Autodesk Fusion 360 part; units mm, degrees
(part 6 of 6)
  spline S1882 degree 3 poles (-65.5883, -15.6255) (-65.5532, -15.6205) (-65.5182, -15.6155) (-65.4821, -15.6104) knots 0 0 0 0 1 1 1 1
  spline S1883 degree 3 poles (-65.4821, -15.6104) (-65.2398, -15.5688) (-65.2398, -15.5688) (-65.135, -15.4302) knots 0 0 0 0 1 1 1 1
  spline S1884 degree 3 poles (-65.135, -15.4302) (-65.0343, -15.1397) (-65.091, -14.7914) (-65.1957, -14.5049) knots 0 0 0 0 1 1 1 1
  spline S1885 degree 3 poles (-65.1957, -14.5049) (-65.2987, -14.382) (-65.405, -14.3558) (-65.5585, -14.321) knots 0 0 0 0 1 1 1 1
  spline S1886 degree 3 poles (-65.5585, -14.321) (-65.627, -14.3026) (-65.627, -14.3026) (-65.6969, -14.2838) knots 0 0 0 0 1 1 1 1
  spline S1887 degree 3 poles (-65.6969, -14.2838) (-65.9478, -14.2203) (-66.2008, -14.1721) (-66.4553, -14.1254) knots 0 0 0 0 1 1 1 1
  spline S1888 degree 3 poles (-66.4553, -14.1254) (-66.8857, -14.0468) (-66.8857, -14.0468) (-67.2221, -13.7882) knots 0 0 0 0 1 1 1 1
  spline S1889 degree 3 poles (-67.2221, -13.7882) (-67.2338, -13.7221) (-67.2455, -13.656) (-67.2575, -13.5879) knots 0 0 0 0 1 1 1 1
  spline S1890 degree 3 poles (-67.2575, -13.5879) (-67.0063, -13.5436) (-66.7551, -13.4993) (-66.4963, -13.4537) knots 0 0 0 0 1 1 1 1
  spline S1891 degree 3 poles (-66.4963, -13.4537) (-66.4997, -13.3198) (-66.5032, -13.186) (-66.5066, -13.0521) knots 0 0 0 0 1 1 1 1
  spline S1892 degree 3 poles (-66.5066, -13.0521) (-66.5107, -12.9269) (-66.5107, -12.9269) (-66.4985, -12.8356) knots 0 0 0 0 1 1 1 1
  spline S1893 degree 3 poles (-66.4985, -12.8356) (-66.495, -12.7075) (-66.5308, -12.5902) (-66.5595, -12.4657) knots 0 0 0 0 1 1 1 1
  spline S1894 degree 3 poles (-66.5595, -12.4657) (-66.6167, -12.177) (-66.5859, -11.9942) (-66.4254, -11.7476) knots 0 0 0 0 1 1 1 1
  spline S1895 degree 3 poles (-66.4254, -11.7476) (-66.3616, -11.6547) (-66.2962, -11.5632) (-66.2298, -11.472) knots 0 0 0 0 1 1 1 1
  spline S1896 degree 3 poles (-66.2298, -11.472) (-66.0403, -11.1911) (-65.8738, -10.8747) (-65.8549, -10.5317) knots 0 0 0 0 1 1 1 1
  spline S1897 degree 3 poles (-65.8549, -10.5317) (-65.8517, -10.4954) (-65.8484, -10.4591) (-65.8451, -10.4217) knots 0 0 0 0 1 1 1 1
  spline S1898 degree 3 poles (-65.8451, -10.4217) (-65.8423, -10.2464) (-65.8489, -10.1305) (-65.972, -9.9994) knots 0 0 0 0 1 1 1 1
  spline S1899 degree 3 poles (-65.972, -9.9994) (-66.0832, -9.9196) (-66.1966, -9.8527) (-66.3167, -9.787) knots 0 0 0 0 1 1 1 1
  spline S1900 degree 3 poles (-66.3167, -9.787) (-66.3519, -9.766) (-66.3871, -9.745) (-66.4234, -9.7234) knots 0 0 0 0 1 1 1 1
  spline S1901 degree 3 poles (-66.4234, -9.7234) (-67.0299, -9.3691) (-67.6639, -9.045) (-68.3125, -8.7758) knots 0 0 0 0 1 1 1 1
  spline S1902 degree 3 poles (-68.3125, -8.7758) (-68.3713, -8.7504) (-68.43, -8.7249) (-68.4886, -8.6994) knots 0 0 0 0 1 1 1 1
  spline S1903 degree 3 poles (-68.4886, -8.6994) (-68.8092, -8.5606) (-69.1312, -8.4289) (-69.4605, -8.3121) knots 0 0 0 0 1 1 1 1
  spline S1904 degree 3 poles (-69.4605, -8.3121) (-69.4898, -8.3016) (-69.519, -8.2912) (-69.5492, -8.2804) knots 0 0 0 0 1 1 1 1
  spline S1905 degree 3 poles (-69.5492, -8.2804) (-69.8961, -8.1602) (-70.2263, -8.1917) (-70.5689, -8.3301) knots 0 0 0 0 1 1 1 1
  spline S1906 degree 3 poles (-70.5689, -8.3301) (-71.0757, -8.6136) (-71.3065, -9.1813) (-71.5588, -9.6756) knots 0 0 0 0 1 1 1 1
  spline S1907 degree 3 poles (-71.5588, -9.6756) (-71.6206, -9.7962) (-71.6842, -9.9157) (-71.7488, -10.0348) knots 0 0 0 0 1 1 1 1
  spline S1908 degree 3 poles (-71.7488, -10.0348) (-71.7661, -10.0671) (-71.7835, -10.0994) (-71.8014, -10.1327) knots 0 0 0 0 1 1 1 1
  spline S1909 degree 3 poles (-71.8014, -10.1327) (-71.857, -10.2311) (-71.857, -10.2311) (-71.9354, -10.3313) knots 0 0 0 0 1 1 1 1
  spline S1910 degree 3 poles (-71.9354, -10.3313) (-72.0284, -10.4725) (-72.0876, -10.6124) (-72.1415, -10.7713) knots 0 0 0 0 1 1 1 1
  spline S1911 degree 3 poles (-72.1415, -10.7713) (-72.152, -10.8016) (-72.1624, -10.8319) (-72.1732, -10.8631) knots 0 0 0 0 1 1 1 1
  spline S1912 degree 3 poles (-72.1732, -10.8631) (-72.3084, -11.2678) (-72.4026, -11.6835) (-72.5002, -12.0984) knots 0 0 0 0 1 1 1 1
  spline S1913 degree 3 poles (-72.5002, -12.0984) (-72.6463, -13.0231) (-72.6463, -13.0231) (-73.0404, -13.8227) knots 0 0 0 0 1 1 1 1
  spline S1914 degree 3 poles (-73.0404, -13.8227) (-73.1439, -13.8634) (-73.2458, -13.891) (-73.3538, -13.9193) knots 0 0 0 0 1 1 1 1
  spline S1915 degree 3 poles (-73.3538, -13.9193) (-73.3286, -13.9617) (-73.3035, -14.0041) (-73.2775, -14.0477) knots 0 0 0 0 1 1 1 1
  spline S1916 degree 3 poles (-73.2775, -14.0477) (-73.1826, -14.2076) (-73.0879, -14.3676) (-72.9931, -14.5276) knots 0 0 0 0 1 1 1 1
  spline S1917 degree 3 poles (-72.9931, -14.5276) (-72.9524, -14.5964) (-72.9117, -14.6651) (-72.8709, -14.7338) knots 0 0 0 0 1 1 1 1
  spline S1918 degree 3 poles (-72.8709, -14.7338) (-72.4098, -15.5103) (-71.9883, -16.2311) (-71.8222, -17.1294) knots 0 0 0 0 1 1 1 1
  spline S1919 degree 3 poles (-71.8222, -17.1294) (-71.814, -17.1724) (-71.8059, -17.2155) (-71.7975, -17.2598) knots 0 0 0 0 1 1 1 1
  spline S1920 degree 3 poles (-71.7975, -17.2598) (-71.7166, -17.7347) (-71.7778, -18.178) (-71.8669, -18.6475) knots 0 0 0 0 1 1 1 1
  spline S1921 degree 3 poles (-71.8669, -18.6475) (-71.8753, -18.6921) (-71.8838, -18.7366) (-71.8925, -18.7825) knots 0 0 0 0 1 1 1 1
  spline S1922 degree 3 poles (-71.8925, -18.7825) (-71.9993, -19.3246) (-72.1479, -19.8096) (-72.438, -20.2844) knots 0 0 0 0 1 1 1 1
  spline S1923 degree 3 poles (-72.438, -20.2844) (-72.4548, -20.3194) (-72.4715, -20.3544) (-72.4888, -20.3905) knots 0 0 0 0 1 1 1 1
  spline S1924 degree 3 poles (-72.4888, -20.3905) (-72.5833, -20.565) (-72.6683, -20.6588) (-72.859, -20.7171) knots 0 0 0 0 1 1 1 1
  spline S1925 degree 3 poles (-72.859, -20.7171) (-73.0033, -20.754) (-73.1488, -20.7807) (-73.2957, -20.8049) knots 0 0 0 0 1 1 1 1
  spline S1926 degree 3 poles (-73.2957, -20.8049) (-73.376, -20.8215) (-73.376, -20.8215) (-73.5135, -20.874) knots 0 0 0 0 1 1 1 1
  spline S1927 degree 3 poles (-73.5135, -20.874) (-73.6824, -20.92) (-73.8082, -20.8944) (-73.9726, -20.8493) knots 0 0 0 0 1 1 1 1
  spline S1928 degree 3 poles (-73.9726, -20.8493) (-74.0026, -20.8414) (-74.0327, -20.8335) (-74.0636, -20.8253) knots 0 0 0 0 1 1 1 1
  spline S1929 degree 3 poles (-74.0636, -20.8253) (-75.2169, -20.508) (-75.8729, -19.7935) (-76.5711, -18.8652) knots 0 0 0 0 1 1 1 1
  spline S1930 degree 3 poles (-76.5711, -18.8652) (-76.6006, -18.8261) (-76.6006, -18.8261) (-76.6307, -18.7863) knots 0 0 0 0 1 1 1 1
  spline S1931 degree 3 poles (-76.6307, -18.7863) (-76.8351, -18.5226) (-76.8351, -18.5226) (-77.0117, -18.2406) knots 0 0 0 0 1 1 1 1
  spline S1932 degree 3 poles (-77.0117, -18.2406) (-77.1093, -18.214) (-77.1093, -18.214) (-77.2261, -18.1958) knots 0 0 0 0 1 1 1 1
  spline S1933 degree 3 poles (-77.2261, -18.1958) (-77.26, -18.1873) (-77.2939, -18.1788) (-77.3288, -18.17) knots 0 0 0 0 1 1 1 1
  spline S1934 degree 3 poles (-77.3288, -18.17) (-77.6049, -18.1231) (-77.8749, -18.1799) (-78.1471, -18.2291) knots 0 0 0 0 1 1 1 1
  spline S1935 degree 3 poles (-78.1471, -18.2291) (-78.1833, -18.2354) (-78.2195, -18.2416) (-78.2568, -18.248) knots 0 0 0 0 1 1 1 1
  spline S1936 degree 3 poles (-78.2568, -18.248) (-78.4722, -18.2863) (-78.6745, -18.3386) (-78.8828, -18.4053) knots 0 0 0 0 1 1 1 1
  spline S1937 degree 3 poles (-78.8828, -18.4053) (-79.2946, -18.5224) (-79.2946, -18.5224) (-79.6968, -18.4301) knots 0 0 0 0 1 1 1 1
  spline S1938 degree 3 poles (-79.6968, -18.4301) (-79.7779, -18.38) (-79.7779, -18.38) (-79.8466, -18.3274) knots 0 0 0 0 1 1 1 1
  spline S1939 degree 3 poles (-79.8466, -18.3274) (-79.8777, -18.3056) (-79.9088, -18.2839) (-79.9408, -18.2614) knots 0 0 0 0 1 1 1 1
  spline S1940 degree 3 poles (-79.9408, -18.2614) (-79.9702, -18.1606) (-79.9702, -18.1606) (-79.9867, -18.0449) knots 0 0 0 0 1 1 1 1
  spline S1941 degree 3 poles (-79.9867, -18.0449) (-79.9933, -18.0061) (-79.9999, -17.9673) (-80.0067, -17.9273) knots 0 0 0 0 1 1 1 1
  spline S1942 degree 3 poles (-80.0067, -17.9273) (-80.0235, -17.8171) (-80.0235, -17.8171) (-79.9997, -17.6935) knots 0 0 0 0 1 1 1 1
  spline S1943 degree 3 poles (-79.9997, -17.6935) (-80.0127, -17.4367) (-80.0653, -17.2516) (-80.2492, -17.0682) knots 0 0 0 0 1 1 1 1
  spline S1944 degree 3 poles (-80.2492, -17.0682) (-80.3329, -17.0032) (-80.4149, -16.9607) (-80.5111, -16.9162) knots 0 0 0 0 1 1 1 1
  spline S1945 degree 3 poles (-80.5111, -16.9162) (-80.7636, -16.7989) (-80.8627, -16.6336) (-80.9708, -16.3835) knots 0 0 0 0 1 1 1 1
  spline S1946 degree 3 poles (-80.9708, -16.3835) (-81.0257, -16.194) (-80.9508, -16.0807) (-80.843, -15.9266) knots 0 0 0 0 1 1 1 1
  spline S1947 degree 3 poles (-61.3294, -20.2671) (-61.263, -20.2962) (-61.263, -20.2962) (-61.1951, -20.326) knots 0 0 0 0 1 1 1 1
  spline S1948 degree 3 poles (-61.1951, -20.326) (-61.2348, -20.333) (-61.2744, -20.34) (-61.3153, -20.3472) knots 0 0 0 0 1 1 1 1
  spline S1949 degree 3 poles (-61.3153, -20.3472) (-61.32, -20.3207) (-61.3246, -20.2943) (-61.3294, -20.2671) knots 0 0 0 0 1 1 1 1
  spline S1950 degree 3 poles (-59.751, 10.372) (-59.6633, 10.465) (-59.5616, 10.5119) (-59.4464, 10.565) knots 0 0 0 0 1 1 1 1
  spline S1951 degree 3 poles (-59.4464, 10.565) (-59.4153, 10.5807) (-59.3843, 10.5964) (-59.3523, 10.6127) knots 0 0 0 0 1 1 1 1
  spline S1952 degree 3 poles (-59.3523, 10.6127) (-59.2858, 10.6462) (-59.219, 10.6791) (-59.152, 10.7115) knots 0 0 0 0 1 1 1 1
  spline S1953 degree 3 poles (-59.152, 10.7115) (-58.977, 10.7962) (-58.8043, 10.8855) (-58.6312, 10.9741) knots 0 0 0 0 1 1 1 1
  spline S1954 degree 3 poles (-58.6312, 10.9741) (-58.5971, 10.9914) (-58.5629, 11.0088) (-58.5277, 11.0266) knots 0 0 0 0 1 1 1 1
  spline S1955 degree 3 poles (-58.5277, 11.0266) (-57.7705, 11.4124) (-57.0352, 11.9023) (-56.4295, 12.5015) knots 0 0 0 0 1 1 1 1
  spline S1956 degree 3 poles (-56.4295, 12.5015) (-56.0056, 12.9201) (-55.4738, 13.0694) (-54.9102, 13.212) knots 0 0 0 0 1 1 1 1
  spline S1957 degree 3 poles (-54.9102, 13.212) (-54.2791, 13.3732) (-53.6906, 13.592) (-53.0958, 13.8587) knots 0 0 0 0 1 1 1 1
  spline S1958 degree 3 poles (-53.0958, 13.8587) (-52.9602, 13.9188) (-52.8245, 13.9787) (-52.6887, 14.0383) knots 0 0 0 0 1 1 1 1
  spline S1959 degree 3 poles (-52.6887, 14.0383) (-52.6043, 14.0754) (-52.52, 14.113) (-52.4359, 14.151) knots 0 0 0 0 1 1 1 1
  spline S1960 degree 3 poles (-52.4359, 14.151) (-52.3984, 14.1676) (-52.3609, 14.1843) (-52.3223, 14.2014) knots 0 0 0 0 1 1 1 1
  spline S1961 degree 3 poles (-52.3223, 14.2014) (-52.2894, 14.2163) (-52.2565, 14.2311) (-52.2226, 14.2464) knots 0 0 0 0 1 1 1 1
  spline S1962 degree 3 poles (-52.2226, 14.2464) (-52.1313, 14.2848) (-52.1313, 14.2848) (-52.0094, 14.2568) knots 0 0 0 0 1 1 1 1
  spline S1963 degree 3 poles (-52.0094, 14.2568) (-52.0534, 14.2314) (-52.0974, 14.206) (-52.1428, 14.1798) knots 0 0 0 0 1 1 1 1
  spline S1964 degree 3 poles (-52.1428, 14.1798) (-52.5791, 13.919) (-52.9072, 13.6269) (-53.2354, 13.2404) knots 0 0 0 0 1 1 1 1
  spline S1965 degree 3 poles (-53.2354, 13.2404) (-53.3211, 13.1403) (-53.4099, 13.0432) (-53.4989, 12.946) knots 0 0 0 0 1 1 1 1
  spline S1966 degree 3 poles (-53.4989, 12.946) (-53.6938, 12.7322) (-53.8771, 12.5123) (-54.0526, 12.2821) knots 0 0 0 0 1 1 1 1
  spline S1967 degree 3 poles (-54.0526, 12.2821) (-54.1106, 12.2071) (-54.1701, 12.136) (-54.233, 12.0652) knots 0 0 0 0 1 1 1 1
  spline S1968 degree 3 poles (-54.233, 12.0652) (-54.3312, 11.9443) (-54.4082, 11.8212) (-54.4872, 11.6874) knots 0 0 0 0 1 1 1 1
  spline S1969 degree 3 poles (-54.4872, 11.6874) (-54.5654, 11.5559) (-54.6458, 11.4259) (-54.7274, 11.2965) knots 0 0 0 0 1 1 1 1
  spline S1970 degree 3 poles (-54.7274, 11.2965) (-54.7428, 11.2721) (-54.7582, 11.2477) (-54.774, 11.2226) knots 0 0 0 0 1 1 1 1
  spline S1971 degree 3 poles (-54.774, 11.2226) (-54.857, 11.093) (-54.9434, 10.9736) (-55.0452, 10.8584) knots 0 0 0 0 1 1 1 1
  spline S1972 degree 3 poles (-55.0452, 10.8584) (-55.2359, 10.6313) (-55.3492, 10.3545) (-55.4744, 10.0881) knots 0 0 0 0 1 1 1 1
  spline S1973 degree 3 poles (-55.4744, 10.0881) (-55.5326, 9.9644) (-55.5924, 9.8415) (-55.6523, 9.7187) knots 0 0 0 0 1 1 1 1
  spline S1974 degree 3 poles (-55.6523, 9.7187) (-55.6804, 9.6603) (-55.6804, 9.6603) (-55.7091, 9.6007) knots 0 0 0 0 1 1 1 1
  spline S1975 degree 3 poles (-55.7091, 9.6007) (-55.7555, 9.5039) (-55.7555, 9.5039) (-55.8229, 9.4123) knots 0 0 0 0 1 1 1 1
  spline S1976 degree 3 poles (-55.8229, 9.4123) (-55.931, 9.3943) (-56.0328, 9.3834) (-56.1419, 9.3767) knots 0 0 0 0 1 1 1 1
  spline S1977 degree 3 poles (-56.1419, 9.3767) (-56.1755, 9.3747) (-56.2092, 9.3726) (-56.2439, 9.3704) knots 0 0 0 0 1 1 1 1
  spline S1978 degree 3 poles (-56.2439, 9.3704) (-56.9302, 9.336) (-57.6315, 9.3267) (-58.2906, 9.5376) knots 0 0 0 0 1 1 1 1
  spline S1979 degree 3 poles (-58.2906, 9.5376) (-58.5865, 9.6318) (-58.8906, 9.6973) (-59.1928, 9.7682) knots 0 0 0 0 1 1 1 1
  spline S1980 degree 3 poles (-59.1928, 9.7682) (-59.2522, 9.7823) (-59.3116, 9.7963) (-59.3711, 9.8104) knots 0 0 0 0 1 1 1 1
  spline S1981 degree 3 poles (-59.3711, 9.8104) (-59.5119, 9.8438) (-59.6527, 9.877) (-59.7935, 9.9101) knots 0 0 0 0 1 1 1 1
  spline S1982 degree 3 poles (-59.7935, 9.9101) (-59.8214, 10.0683) (-59.8022, 10.2204) (-59.751, 10.372) knots 0 0 0 0 1 1 1 1
  line L6 (-50.8593, 14.9966) -> (-50.9465, 15.0225)
  line L7 (-50.7862, 15.0507) -> (-50.8734, 15.0767)
  spline S1983 degree 3 poles (-29.2882, 12.6041) (-28.8697, 12.7557) (-28.5896, 12.7131) (-28.1934, 12.5283) knots 0 0 0 0 1 1 1 1
  spline S1984 degree 3 poles (-28.1934, 12.5283) (-28.0851, 12.4763) (-27.9778, 12.4225) (-27.8706, 12.3684) knots 0 0 0 0 1 1 1 1
  spline S1985 degree 3 poles (-27.8706, 12.3684) (-27.7226, 12.2949) (-27.5716, 12.228) (-27.4211, 12.1599) knots 0 0 0 0 1 1 1 1
  spline S1986 degree 3 poles (-27.4211, 12.1599) (-27.3957, 12.147) (-27.3703, 12.134) (-27.3442, 12.1207) knots 0 0 0 0 1 1 1 1
  spline S1987 degree 3 poles (-27.3442, 12.1207) (-27.3418, 12.1075) (-27.3395, 12.0943) (-27.3371, 12.0806) knots 0 0 0 0 1 1 1 1
  spline S1988 degree 3 poles (-27.3371, 12.0806) (-27.3612, 12.0758) (-27.3853, 12.071) (-27.4102, 12.0661) knots 0 0 0 0 1 1 1 1
  spline S1989 degree 3 poles (-27.4102, 12.0661) (-27.6928, 11.9997) (-27.879, 11.8794) (-28.1005, 11.6956) knots 0 0 0 0 1 1 1 1
  spline S1990 degree 3 poles (-28.1005, 11.6956) (-28.1317, 11.6706) (-28.1628, 11.6456) (-28.1949, 11.6198) knots 0 0 0 0 1 1 1 1
  spline S1991 degree 3 poles (-28.1949, 11.6198) (-28.2708, 11.5588) (-28.3462, 11.4972) (-28.4212, 11.4351) knots 0 0 0 0 1 1 1 1
  spline S1992 degree 3 poles (-28.4212, 11.4351) (-28.5203, 11.5389) (-28.5593, 11.6131) (-28.6197, 11.7409) knots 0 0 0 0 1 1 1 1
  spline S1993 degree 3 poles (-28.6197, 11.7409) (-28.7463, 11.9829) (-28.9129, 12.1609) (-29.1051, 12.3513) knots 0 0 0 0 1 1 1 1
  spline S1994 degree 3 poles (-29.1051, 12.3513) (-29.2274, 12.4594) (-29.2274, 12.4594) (-29.2882, 12.6041) knots 0 0 0 0 1 1 1 1
  spline S1995 degree 3 poles (-8.3515, -3.8776) (-8.3386, -3.8501) (-8.3257, -3.8226) (-8.3125, -3.7942) knots 0 0 0 0 1 1 1 1
  spline S1996 degree 3 poles (-8.3125, -3.7942) (-8.2806, -3.7262) (-8.2484, -3.6583) (-8.2162, -3.5904) knots 0 0 0 0 1 1 1 1
  spline S1997 degree 3 poles (-8.2162, -3.5904) (-8.1894, -3.6266) (-8.1894, -3.6266) (-8.1621, -3.6635) knots 0 0 0 0 1 1 1 1
  spline S1998 degree 3 poles (-8.1621, -3.6635) (-8.1884, -3.7667) (-8.1884, -3.7667) (-8.2348, -3.8803) knots 0 0 0 0 1 1 1 1
  spline S1999 degree 3 poles (-8.2348, -3.8803) (-8.2495, -3.919) (-8.2641, -3.9577) (-8.2792, -3.9976) knots 0 0 0 0 1 1 1 1
  spline S2000 degree 3 poles (-8.2792, -3.9976) (-8.3311, -4.105) (-8.3848, -4.1735) (-8.4708, -4.2549) knots 0 0 0 0 1 1 1 1
  spline S2001 degree 3 poles (-8.4708, -4.2549) (-8.495, -4.1179) (-8.4095, -3.9996) (-8.3515, -3.8776) knots 0 0 0 0 1 1 1 1
  spline S2002 degree 3 poles (-21.8258, -8.6338) (-21.2854, -9.6912) (-19.7141, -10.0697) (-18.6621, -10.4138) knots 0 0 0 0 1 1 1 1
  spline S2003 degree 3 poles (-18.6621, -10.4138) (-17.9941, -10.6297) (-17.3212, -10.8297) (-16.6476, -11.0274) knots 0 0 0 0 1 1 1 1
  spline S2004 degree 3 poles (-16.6476, -11.0274) (-16.588, -11.045) (-16.5284, -11.0625) (-16.4689, -11.0801) knots 0 0 0 0 1 1 1 1
  spline S2005 degree 3 poles (-16.4689, -11.0801) (-16.4402, -11.0885) (-16.4115, -11.0969) (-16.382, -11.1055) knots 0 0 0 0 1 1 1 1
  spline S2006 degree 3 poles (-16.382, -11.1055) (-16.2422, -11.1468) (-16.1039, -11.1905) (-15.9666, -11.2396) knots 0 0 0 0 1 1 1 1
  spline S2007 degree 3 poles (-15.9666, -11.2396) (-15.8908, -11.2665) (-15.8908, -11.2665) (-15.8135, -11.294) knots 0 0 0 0 1 1 1 1
  spline S2008 degree 3 poles (-15.8135, -11.294) (-15.7691, -11.3105) (-15.7248, -11.327) (-15.6791, -11.344) knots 0 0 0 0 1 1 1 1
  spline S2009 degree 3 poles (-15.6791, -11.344) (-15.5418, -11.3747) (-15.489, -11.3611) (-15.367, -11.2952) knots 0 0 0 0 1 1 1 1
  spline S2010 degree 3 poles (-15.367, -11.2952) (-14.9346, -10.9867) (-14.5857, -10.5916) (-14.2319, -10.1995) knots 0 0 0 0 1 1 1 1
  spline S2011 degree 3 poles (-14.2319, -10.1995) (-13.5392, -9.4271) (-13.5392, -9.4271) (-12.6736, -8.8685) knots 0 0 0 0 1 1 1 1
  spline S2012 degree 3 poles (-12.6736, -8.8685) (-12.49, -8.7721) (-12.3953, -8.6319) (-12.2747, -8.4667) knots 0 0 0 0 1 1 1 1
  spline S2013 degree 3 poles (-12.2747, -8.4667) (-12.1495, -8.3018) (-12.0022, -8.1585) (-11.8565, -8.0119) knots 0 0 0 0 1 1 1 1
  spline S2014 degree 3 poles (-11.8565, -8.0119) (-11.6201, -7.7723) (-11.4014, -7.5307) (-11.2048, -7.2567) knots 0 0 0 0 1 1 1 1
  spline S2015 degree 3 poles (-11.2048, -7.2567) (-11.1876, -7.233) (-11.1703, -7.2093) (-11.1525, -7.1849) knots 0 0 0 0 1 1 1 1
  spline S2016 degree 3 poles (-11.1525, -7.1849) (-11.0963, -7.1076) (-11.0405, -7.0299) (-10.9849, -6.952) knots 0 0 0 0 1 1 1 1
  spline S2017 degree 3 poles (-10.9849, -6.952) (-10.9672, -6.9274) (-10.9494, -6.9027) (-10.9312, -6.8773) knots 0 0 0 0 1 1 1 1
  spline S2018 degree 3 poles (-10.9312, -6.8773) (-10.8885, -6.8166) (-10.8484, -6.754) (-10.8088, -6.6912) knots 0 0 0 0 1 1 1 1
  spline S2019 degree 3 poles (-10.8088, -6.6912) (-10.8135, -6.6648) (-10.8182, -6.6383) (-10.823, -6.6111) knots 0 0 0 0 1 1 1 1
  spline S2020 degree 3 poles (-10.823, -6.6111) (-10.9778, -6.6113) (-11.1325, -6.6121) (-11.2873, -6.6129) knots 0 0 0 0 1 1 1 1
  spline S2021 degree 3 poles (-11.2873, -6.6129) (-11.352, -6.613) (-11.352, -6.613) (-11.418, -6.6131) knots 0 0 0 0 1 1 1 1
  spline S2022 degree 3 poles (-11.418, -6.6131) (-11.4826, -6.6136) (-11.4826, -6.6136) (-11.5486, -6.614) knots 0 0 0 0 1 1 1 1
  spline S2023 degree 3 poles (-11.5486, -6.614) (-11.5875, -6.6141) (-11.6264, -6.6143) (-11.6665, -6.6144) knots 0 0 0 0 1 1 1 1
  spline S2024 degree 3 poles (-11.6665, -6.6144) (-12.1146, -6.6326) (-12.5512, -6.7031) (-12.9919, -6.7815) knots 0 0 0 0 1 1 1 1
  spline S2025 degree 3 poles (-12.9919, -6.7815) (-13.0579, -6.7931) (-13.124, -6.8047) (-13.19, -6.8163) knots 0 0 0 0 1 1 1 1
  spline S2026 degree 3 poles (-13.19, -6.8163) (-13.3278, -6.8405) (-13.4656, -6.8649) (-13.6033, -6.8894) knots 0 0 0 0 1 1 1 1
  spline S2027 degree 3 poles (-13.6033, -6.8894) (-13.778, -6.9204) (-13.9527, -6.9511) (-14.1275, -6.9817) knots 0 0 0 0 1 1 1 1
  spline S2028 degree 3 poles (-14.1275, -6.9817) (-14.2637, -7.0056) (-14.4, -7.0296) (-14.5362, -7.0538) knots 0 0 0 0 1 1 1 1
  spline S2029 degree 3 poles (-14.5362, -7.0538) (-14.6005, -7.0651) (-14.6649, -7.0764) (-14.7292, -7.0877) knots 0 0 0 0 1 1 1 1
  spline S2030 degree 3 poles (-14.7292, -7.0877) (-15.0383, -7.1418) (-15.3443, -7.1996) (-15.6489, -7.2759) knots 0 0 0 0 1 1 1 1
  spline S2031 degree 3 poles (-15.6489, -7.2759) (-16.021, -7.3683) (-16.3969, -7.4356) (-16.7741, -7.5034) knots 0 0 0 0 1 1 1 1
  spline S2032 degree 3 poles (-16.7741, -7.5034) (-16.9055, -7.5271) (-17.0368, -7.5511) (-17.1681, -7.5751) knots 0 0 0 0 1 1 1 1
  spline S2033 degree 3 poles (-17.1681, -7.5751) (-17.5411, -7.6434) (-17.9141, -7.7114) (-18.2872, -7.7786) knots 0 0 0 0 1 1 1 1
  spline S2034 degree 3 poles (-18.2872, -7.7786) (-20.2851, -8.1387) (-20.2851, -8.1387) (-21.239, -8.4477) knots 0 0 0 0 1 1 1 1
  spline S2035 degree 3 poles (-21.239, -8.4477) (-21.3066, -8.4688) (-21.3742, -8.4898) (-21.4418, -8.5107) knots 0 0 0 0 1 1 1 1
  spline S2036 degree 3 poles (-21.4418, -8.5107) (-21.5702, -8.5505) (-21.6982, -8.5915) (-21.8258, -8.6338) knots 0 0 0 0 1 1 1 1
  spline S2037 degree 3 poles (-20.2846, -8.9403) (-19.8892, -8.8299) (-19.4907, -8.7519) (-19.0871, -8.6784) knots 0 0 0 0 1 1 1 1
  spline S2038 degree 3 poles (-19.0871, -8.6784) (-18.9719, -8.6574) (-18.8567, -8.6361) (-18.7416, -8.6149) knots 0 0 0 0 1 1 1 1
  spline S2039 degree 3 poles (-18.7416, -8.6149) (-18.5768, -8.5844) (-18.4119, -8.554) (-18.2471, -8.5237) knots 0 0 0 0 1 1 1 1
  spline S2040 degree 3 poles (-18.2471, -8.5237) (-16.8732, -8.2708) (-15.5027, -8.0084) (-14.1374, -7.713) knots 0 0 0 0 1 1 1 1
  spline S2041 degree 3 poles (-14.1374, -7.713) (-13.5391, -7.5836) (-12.9449, -7.4619) (-12.3336, -7.4144) knots 0 0 0 0 1 1 1 1
  spline S2042 degree 3 poles (-12.3336, -7.4144) (-12.4282, -7.5573) (-12.5326, -7.677) (-12.6531, -7.7987) knots 0 0 0 0 1 1 1 1
  spline S2043 degree 3 poles (-12.6531, -7.7987) (-12.7577, -7.9044) (-12.8551, -8.008) (-12.9472, -8.125) knots 0 0 0 0 1 1 1 1
  spline S2044 degree 3 poles (-12.9472, -8.125) (-13.0634, -8.2533) (-13.1826, -8.3271) (-13.3333, -8.4065) knots 0 0 0 0 1 1 1 1
  spline S2045 degree 3 poles (-13.3333, -8.4065) (-13.9324, -8.7442) (-14.363, -9.2406) (-14.813, -9.7517) knots 0 0 0 0 1 1 1 1
  spline S2046 degree 3 poles (-14.813, -9.7517) (-14.9284, -9.8819) (-15.0445, -10.0109) (-15.1642, -10.1372) knots 0 0 0 0 1 1 1 1
  spline S2047 degree 3 poles (-15.1642, -10.1372) (-15.2631, -10.2442) (-15.2631, -10.2442) (-15.3414, -10.3514) knots 0 0 0 0 1 1 1 1
  spline S2048 degree 3 poles (-15.3414, -10.3514) (-15.432, -10.4604) (-15.4865, -10.5096) (-15.6214, -10.5552) knots 0 0 0 0 1 1 1 1
  spline S2049 degree 3 poles (-15.6214, -10.5552) (-15.8636, -10.5279) (-16.0834, -10.4521) (-16.3132, -10.3731) knots 0 0 0 0 1 1 1 1
  spline S2050 degree 3 poles (-16.3132, -10.3731) (-16.4601, -10.3242) (-16.608, -10.2803) (-16.7567, -10.2374) knots 0 0 0 0 1 1 1 1
  spline S2051 degree 3 poles (-16.7567, -10.2374) (-17.417, -10.0467) (-18.0716, -9.8426) (-18.72, -9.6145) knots 0 0 0 0 1 1 1 1
  spline S2052 degree 3 poles (-18.72, -9.6145) (-18.7568, -9.6016) (-18.7936, -9.5888) (-18.8315, -9.5755) knots 0 0 0 0 1 1 1 1
  spline S2053 degree 3 poles (-18.8315, -9.5755) (-19.207, -9.4434) (-19.5785, -9.3047) (-19.9437, -9.1461) knots 0 0 0 0 1 1 1 1
  spline S2054 degree 3 poles (-19.9437, -9.1461) (-19.9721, -9.1339) (-20.0004, -9.1216) (-20.0296, -9.109) knots 0 0 0 0 1 1 1 1
  spline S2055 degree 3 poles (-20.0296, -9.109) (-20.1747, -9.0482) (-20.1747, -9.0482) (-20.2846, -8.9403) knots 0 0 0 0 1 1 1 1
  spline S2056 degree 3 poles (-52.8685, -12.4965) (-52.0897, -12.6031) (-51.4196, -12.4442) (-50.6991, -12.1468) knots 0 0 0 0 1 1 1 1
  spline S2057 degree 3 poles (-50.6991, -12.1468) (-50.264, -11.9695) (-49.8583, -11.8968) (-49.3895, -11.8817) knots 0 0 0 0 1 1 1 1
  spline S2058 degree 3 poles (-49.3895, -11.8817) (-48.9966, -11.8669) (-48.61, -11.8138) (-48.2207, -11.7608) knots 0 0 0 0 1 1 1 1
  spline S2059 degree 3 poles (-48.2207, -11.7608) (-47.8681, -11.7131) (-47.5192, -11.6762) (-47.1631, -11.6713) knots 0 0 0 0 1 1 1 1
  spline S2060 degree 3 poles (-47.1631, -11.6713) (-47.1336, -11.6708) (-47.1041, -11.6703) (-47.0737, -11.6698) knots 0 0 0 0 1 1 1 1
  spline S2061 degree 3 poles (-47.0737, -11.6698) (-46.7465, -11.6693) (-46.3684, -11.7103) (-46.0761, -11.8624) knots 0 0 0 0 1 1 1 1
  spline S2062 degree 3 poles (-46.0761, -11.8624) (-45.9778, -11.9107) (-45.9228, -11.9082) (-45.8145, -11.9007) knots 0 0 0 0 1 1 1 1
  spline S2063 degree 3 poles (-45.8145, -11.9007) (-45.5459, -11.8991) (-45.3117, -11.9909) (-45.0616, -12.0792) knots 0 0 0 0 1 1 1 1
  spline S2064 degree 3 poles (-45.0616, -12.0792) (-44.8559, -12.1495) (-44.7226, -12.1521) (-44.5123, -12.097) knots 0 0 0 0 1 1 1 1
  spline S2065 degree 3 poles (-44.5123, -12.097) (-44.2631, -11.9693) (-44.0986, -11.7687) (-43.9961, -11.5103) knots 0 0 0 0 1 1 1 1
  spline S2066 degree 3 poles (-43.9961, -11.5103) (-43.9224, -11.1796) (-43.8939, -10.8417) (-43.871, -10.504) knots 0 0 0 0 1 1 1 1
  spline S2067 degree 3 poles (-43.871, -10.504) (-43.8624, -10.4021) (-43.8624, -10.4021) (-43.8004, -10.2779) knots 0 0 0 0 1 1 1 1
  spline S2068 degree 3 poles (-43.8004, -10.2779) (-43.8092, -10.1198) (-43.8465, -9.9855) (-43.9181, -9.8443) knots 0 0 0 0 1 1 1 1
  spline S2069 degree 3 poles (-43.9181, -9.8443) (-44.2755, -9.5318) (-44.851, -9.4764) (-45.3061, -9.4694) knots 0 0 0 0 1 1 1 1
  spline S2070 degree 3 poles (-45.3061, -9.4694) (-45.4662, -9.4817) (-45.6217, -9.5074) (-45.7794, -9.5374) knots 0 0 0 0 1 1 1 1
  spline S2071 degree 3 poles (-45.7794, -9.5374) (-45.8224, -9.5452) (-45.8654, -9.553) (-45.9097, -9.5611) knots 0 0 0 0 1 1 1 1
  spline S2072 degree 3 poles (-45.9097, -9.5611) (-46.2492, -9.6265) (-46.5733, -9.7233) (-46.9016, -9.83) knots 0 0 0 0 1 1 1 1
  spline S2073 degree 3 poles (-46.9016, -9.83) (-47.4991, -10.0209) (-48.0848, -10.1241) (-48.7113, -10.0699) knots 0 0 0 0 1 1 1 1
  spline S2074 degree 3 poles (-48.7113, -10.0699) (-49.725, -10.0026) (-50.5529, -10.4397) (-51.412, -10.9178) knots 0 0 0 0 1 1 1 1
  spline S2075 degree 3 poles (-51.412, -10.9178) (-51.9691, -11.2376) (-51.9691, -11.2376) (-52.5617, -11.4804) knots 0 0 0 0 1 1 1 1
  spline S2076 degree 3 poles (-52.5617, -11.4804) (-52.6304, -11.5044) (-52.6304, -11.5044) (-52.6634, -11.5516) knots 0 0 0 0 1 1 1 1
  spline S2077 degree 3 poles (-52.6634, -11.5516) (-52.6532, -11.6186) (-52.6415, -11.6854) (-52.628, -11.7519) knots 0 0 0 0 1 1 1 1
  spline S2078 degree 3 poles (-52.628, -11.7519) (-52.7074, -11.7658) (-52.7867, -11.7798) (-52.8684, -11.7942) knots 0 0 0 0 1 1 1 1
  spline S2079 degree 3 poles (-52.8684, -11.7942) (-52.8726, -11.8887) (-52.8765, -11.9832) (-52.8804, -12.0778) knots 0 0 0 0 1 1 1 1
  spline S2080 degree 3 poles (-52.8804, -12.0778) (-52.8837, -12.1567) (-52.8837, -12.1567) (-52.8871, -12.2372) knots 0 0 0 0 1 1 1 1
  spline S2081 degree 3 poles (-52.8871, -12.2372) (-52.8897, -12.3763) (-52.8897, -12.3763) (-52.8685, -12.4965) knots 0 0 0 0 1 1 1 1
  spline S2082 degree 3 poles (-50.3728, -11.189) (-49.7763, -10.9024) (-49.2643, -10.7643) (-48.6006, -10.8145) knots 0 0 0 0 1 1 1 1
  spline S2083 degree 3 poles (-48.6006, -10.8145) (-47.8499, -10.8686) (-47.154, -10.6753) (-46.4412, -10.4578) knots 0 0 0 0 1 1 1 1
  spline S2084 degree 3 poles (-46.4412, -10.4578) (-45.8156, -10.2684) (-45.2693, -10.1602) (-44.6228, -10.299) knots 0 0 0 0 1 1 1 1
  spline S2085 degree 3 poles (-44.6228, -10.299) (-44.6249, -10.4252) (-44.6279, -10.5513) (-44.631, -10.6774) knots 0 0 0 0 1 1 1 1
  spline S2086 degree 3 poles (-44.631, -10.6774) (-44.6318, -10.7306) (-44.6318, -10.7306) (-44.6327, -10.7848) knots 0 0 0 0 1 1 1 1
  spline S2087 degree 3 poles (-44.6327, -10.7848) (-44.6381, -10.9862) (-44.6577, -11.1582) (-44.7266, -11.35) knots 0 0 0 0 1 1 1 1
  spline S2088 degree 3 poles (-44.7266, -11.35) (-44.9081, -11.3566) (-45.0537, -11.313) (-45.2258, -11.2573) knots 0 0 0 0 1 1 1 1
  spline S2089 degree 3 poles (-45.2258, -11.2573) (-45.439, -11.1904) (-45.6418, -11.1455) (-45.8645, -11.1268) knots 0 0 0 0 1 1 1 1
  spline S2090 degree 3 poles (-45.8645, -11.1268) (-45.9778, -11.1127) (-46.0814, -11.0846) (-46.1912, -11.0532) knots 0 0 0 0 1 1 1 1
  spline S2091 degree 3 poles (-46.1912, -11.0532) (-46.9827, -10.842) (-47.8002, -10.9782) (-48.5992, -11.0739) knots 0 0 0 0 1 1 1 1
  spline S2092 degree 3 poles (-48.5992, -11.0739) (-48.9126, -11.1105) (-49.223, -11.1322) (-49.5383, -11.143) knots 0 0 0 0 1 1 1 1
  spline S2093 degree 3 poles (-49.5383, -11.143) (-49.7136, -11.1505) (-49.8862, -11.168) (-50.0601, -11.1906) knots 0 0 0 0 1 1 1 1
  spline S2094 degree 3 poles (-50.0601, -11.1906) (-50.0902, -11.1943) (-50.1202, -11.198) (-50.1512, -11.2018) knots 0 0 0 0 1 1 1 1
  spline S2095 degree 3 poles (-50.1512, -11.2018) (-50.2227, -11.2107) (-50.2942, -11.2198) (-50.3657, -11.229) knots 0 0 0 0 1 1 1 1
  spline S2096 degree 3 poles (-50.3657, -11.229) (-50.3681, -11.2158) (-50.3704, -11.2026) (-50.3728, -11.189) knots 0 0 0 0 1 1 1 1
  spline S2097 degree 3 poles (-38.3714, 12.4006) (-38.3152, 12.3122) (-38.2526, 12.2703) (-38.1649, 12.2135) knots 0 0 0 0 1 1 1 1
  spline S2098 degree 3 poles (-38.1649, 12.2135) (-38.0595, 12.1447) (-37.9847, 12.0872) (-37.8966, 11.9949) knots 0 0 0 0 1 1 1 1
  spline S2099 degree 3 poles (-37.8966, 11.9949) (-37.7625, 12.0468) (-37.6624, 12.121) (-37.5502, 12.2104) knots 0 0 0 0 1 1 1 1
  spline S2100 degree 3 poles (-37.5502, 12.2104) (-37.5123, 12.2405) (-37.4744, 12.2706) (-37.4353, 12.3016) knots 0 0 0 0 1 1 1 1
  spline S2101 degree 3 poles (-37.4353, 12.3016) (-37.3947, 12.3341) (-37.3541, 12.3666) (-37.3123, 12.4) knots 0 0 0 0 1 1 1 1
  spline S2102 degree 3 poles (-37.3123, 12.4) (-37.2697, 12.4339) (-37.2271, 12.4677) (-37.1846, 12.5015) knots 0 0 0 0 1 1 1 1
  spline S2103 degree 3 poles (-37.1846, 12.5015) (-36.9862, 12.6591) (-36.7885, 12.8175) (-36.5907, 12.976) knots 0 0 0 0 1 1 1 1
  spline S2104 degree 3 poles (-36.5907, 12.976) (-36.5258, 13.028) (-36.4608, 13.0801) (-36.3958, 13.1322) knots 0 0 0 0 1 1 1 1
  spline S2105 degree 3 poles (-36.3958, 13.1322) (-36.364, 13.1577) (-36.3322, 13.1831) (-36.2994, 13.2094) knots 0 0 0 0 1 1 1 1
  spline S2106 degree 3 poles (-36.2994, 13.2094) (-36.0202, 13.4326) (-35.7372, 13.6508) (-35.453, 13.8676) knots 0 0 0 0 1 1 1 1
  spline S2107 degree 3 poles (-35.453, 13.8676) (-35.2465, 14.0253) (-35.043, 14.186) (-34.8422, 14.351) knots 0 0 0 0 1 1 1 1
  spline S2108 degree 3 poles (-34.8422, 14.351) (-34.9389, 14.533) (-35.0736, 14.6533) (-35.2242, 14.7897) knots 0 0 0 0 1 1 1 1
  spline S2109 degree 3 poles (-35.2242, 14.7897) (-35.5152, 15.0577) (-35.7966, 15.3339) (-36.0762, 15.6137) knots 0 0 0 0 1 1 1 1
  spline S2110 degree 3 poles (-36.0762, 15.6137) (-36.1537, 15.6911) (-36.2315, 15.7681) (-36.3094, 15.845) knots 0 0 0 0 1 1 1 1
  spline S2111 degree 3 poles (-36.3094, 15.845) (-36.5971, 16.1291) (-36.8813, 16.4155) (-37.1583, 16.7102) knots 0 0 0 0 1 1 1 1
  spline S2112 degree 3 poles (-37.1583, 16.7102) (-37.2505, 16.5948) (-37.2866, 16.4878) (-37.3243, 16.3456) knots 0 0 0 0 1 1 1 1
  spline S2113 degree 3 poles (-37.3243, 16.3456) (-37.3428, 16.2765) (-37.3428, 16.2765) (-37.3616, 16.2059) knots 0 0 0 0 1 1 1 1
  spline S2114 degree 3 poles (-37.3616, 16.2059) (-37.3747, 16.1554) (-37.3878, 16.1049) (-37.4013, 16.0529) knots 0 0 0 0 1 1 1 1
  spline S2115 degree 3 poles (-37.4013, 16.0529) (-37.4154, 15.9995) (-37.4295, 15.9461) (-37.4435, 15.8927) knots 0 0 0 0 1 1 1 1
  spline S2116 degree 3 poles (-37.4435, 15.8927) (-37.5613, 15.4423) (-37.6679, 14.9894) (-37.7741, 14.5362) knots 0 0 0 0 1 1 1 1
  spline S2117 degree 3 poles (-37.7741, 14.5362) (-37.9259, 13.8897) (-37.9259, 13.8897) (-38.1023, 13.2495) knots 0 0 0 0 1 1 1 1
  spline S2118 degree 3 poles (-38.1023, 13.2495) (-38.1117, 13.2174) (-38.1212, 13.1854) (-38.1309, 13.1523) knots 0 0 0 0 1 1 1 1
  spline S2119 degree 3 poles (-38.1309, 13.1523) (-38.193, 12.9506) (-38.2739, 12.7645) (-38.3682, 12.5755) knots 0 0 0 0 1 1 1 1
  spline S2120 degree 3 poles (-38.3682, 12.5755) (-38.3961, 12.4851) (-38.3961, 12.4851) (-38.3714, 12.4006) knots 0 0 0 0 1 1 1 1
  spline S2121 degree 3 poles (-37.2216, 13.6788) (-37.21, 13.7302) (-37.21, 13.7302) (-37.1981, 13.7827) knots 0 0 0 0 1 1 1 1
  spline S2122 degree 3 poles (-37.1981, 13.7827) (-37.1896, 13.8198) (-37.181, 13.8569) (-37.1722, 13.8952) knots 0 0 0 0 1 1 1 1
  spline S2123 degree 3 poles (-37.1722, 13.8952) (-37.1635, 13.9331) (-37.1548, 13.9711) (-37.1459, 14.0103) knots 0 0 0 0 1 1 1 1
  spline S2124 degree 3 poles (-37.1459, 14.0103) (-37.1274, 14.0907) (-37.1089, 14.1711) (-37.0902, 14.2514) knots 0 0 0 0 1 1 1 1
  spline S2125 degree 3 poles (-37.0902, 14.2514) (-37.0617, 14.3748) (-37.0337, 14.4983) (-37.0057, 14.6218) knots 0 0 0 0 1 1 1 1
  spline S2126 degree 3 poles (-37.0057, 14.6218) (-36.9877, 14.6998) (-36.9697, 14.7777) (-36.9517, 14.8557) knots 0 0 0 0 1 1 1 1
  spline S2127 degree 3 poles (-36.9517, 14.8557) (-36.9433, 14.8928) (-36.935, 14.93) (-36.9263, 14.9683) knots 0 0 0 0 1 1 1 1
  spline S2128 degree 3 poles (-36.9263, 14.9683) (-36.9183, 15.0025) (-36.9103, 15.0367) (-36.902, 15.072) knots 0 0 0 0 1 1 1 1
  spline S2129 degree 3 poles (-36.902, 15.072) (-36.8951, 15.1022) (-36.8881, 15.1324) (-36.8809, 15.1636) knots 0 0 0 0 1 1 1 1
  spline S2130 degree 3 poles (-36.8809, 15.1636) (-36.8622, 15.2419) (-36.8622, 15.2419) (-36.7839, 15.2892) knots 0 0 0 0 1 1 1 1
  spline S2131 degree 3 poles (-36.7839, 15.2892) (-36.6879, 15.1942) (-36.592, 15.0993) (-36.4961, 15.0043) knots 0 0 0 0 1 1 1 1
  spline S2132 degree 3 poles (-36.4961, 15.0043) (-36.4692, 14.9776) (-36.4422, 14.951) (-36.4144, 14.9235) knots 0 0 0 0 1 1 1 1
  spline S2133 degree 3 poles (-36.4144, 14.9235) (-36.3371, 14.8468) (-36.26, 14.7699) (-36.183, 14.6929) knots 0 0 0 0 1 1 1 1
  spline S2134 degree 3 poles (-36.183, 14.6929) (-36.1618, 14.6718) (-36.1406, 14.6507) (-36.1188, 14.6289) knots 0 0 0 0 1 1 1 1
  spline S2135 degree 3 poles (-36.1188, 14.6289) (-36.0149, 14.5305) (-36.0149, 14.5305) (-35.9663, 14.4006) knots 0 0 0 0 1 1 1 1
  spline S2136 degree 3 poles (-35.9663, 14.4006) (-36.1126, 14.2888) (-36.259, 14.1771) (-36.4053, 14.0653) knots 0 0 0 0 1 1 1 1
  spline S2137 degree 3 poles (-36.4053, 14.0653) (-36.4551, 14.0273) (-36.5048, 13.9894) (-36.5545, 13.9514) knots 0 0 0 0 1 1 1 1
  spline S2138 degree 3 poles (-36.5545, 13.9514) (-36.6262, 13.8966) (-36.698, 13.8418) (-36.7697, 13.787) knots 0 0 0 0 1 1 1 1
  spline S2139 degree 3 poles (-36.7697, 13.787) (-36.7917, 13.7702) (-36.8137, 13.7534) (-36.8363, 13.7361) knots 0 0 0 0 1 1 1 1
  spline S2140 degree 3 poles (-36.8363, 13.7361) (-36.9705, 13.6337) (-37.1055, 13.5326) (-37.2413, 13.4323) knots 0 0 0 0 1 1 1 1
  spline S2141 degree 3 poles (-37.2413, 13.4323) (-37.2579, 13.5266) (-37.2428, 13.5855) (-37.2216, 13.6788) knots 0 0 0 0 1 1 1 1
  spline S2142 degree 3 poles (-61.6523, -20.0761) (-61.6114, -20.1916) (-61.6114, -20.1916) (-61.5698, -20.3094) knots 0 0 0 0 1 1 1 1
  spline S2143 degree 3 poles (-61.5698, -20.3094) (-61.4882, -20.3087) (-61.4065, -20.3079) (-61.3224, -20.3071) knots 0 0 0 0 1 1 1 1
  spline S2144 degree 3 poles (-61.3224, -20.3071) (-61.3161, -20.2651) (-61.3099, -20.2231) (-61.3035, -20.1799) knots 0 0 0 0 1 1 1 1
  spline S2145 degree 3 poles (-61.3035, -20.1799) (-61.5621, -20.0602) (-61.5621, -20.0602) (-61.6523, -20.0761) knots 0 0 0 0 1 1 1 1
  line L8 (-52.4648, -1) -> (-47, -1)
  line L9 (-47, -1) -> (-10.3014, -0.9013)
  circle A4 centre (-5, -5) radius 4.5014
  constraint coincident S1306 L8.start
  constraint parallel L0 L8
  constraint concentric A0 A4
  constraint coincident S1603.end S1604.start
extrude "Extrude4" cut sketch "Sketch4" against normal blind 0.25 contours S1644 S1645 S1646 S1647 S1648 S1649 S1650 S1651 S1652 S1653 S1654 S1655 S1656 S1657 S1658 S1659 S1660 S1661 S1662 S1663 S1664 S1665 A4 | S1242 S1243 S1244 S1245 S1246 S1247 S1248 S1249 S1250 S1251 S1252 S1253 S1254 S1255 S1256 S1257 S1258 S1259 S1260 S1261 S1262 S1263 S1264 S1265 S1266 S1267 S1268 S1269 S1270 S1271 S1272 S1273 S1274 S1275 S1276 S1277 S1278 S1279 S1280 S1281 S1282 S1283 S1284 S1285 S1286 S1287 S1288 S1289 S1290 S1291 S1292 S1293 S1294 S1295 S1296 S1297 S1298 S1299 S1300 S1301 S1302 S1303 S1304 S1305 S1306 S1604 S1605 S1606 S1607 S1608 S1609 S1610 S1611 S1612 S1613 S1614 S1615 S1616 S1617 S1618 S1619 S1620 S1621 S1622 S1623 S1624 S1625 S1626 S1627 S1628 S1629 S1630 S1631 S1632 S1633 S1634 S1635 S1636 S1637 S1638 S1639 S1640 S1641 S1642 S1643 S1644 S1665 S1666 S1667 S1668 S1669 S1670 S1671 S1672 S1673 S1674 S1675 S1676 S1677 S1678 S1679 S1680 S1681 S1682 S1683 S1684 S1685 S1686 S1687 S1688 S1689 S1690 S1691 S1692 S1693 S1694 S1695 S1696 S1697 S1698 S1699 S1700 S1701 S1702 S1703 S1704 S1705 S1706 S1707 S1708 S1709 S1710 S1711 S1712 S1713 S1714 S1715 S1716 S1717 S1718 S1719 S1720 S1721 S1722 S1723 S1724 S1725 S1726 S1727 S1728 S1729 S1730 S1731 S1732 S1733 S1734 S1735 S1736 S1737 S1738 S1739 S1740 S1741 S1742 S1743 S1744 S1745 S1746 S1747 S1748 S1749 S1750 S1751 S1752 S1753 S1754 S1755 S1756 S1757 S1758 S1759 S1760 S1761 S1762 S1763 S1764 S1765 S1766 S1767 S1768 S1769 S1770 S1771 S1772 S1773 S1774 S1775 S1776 S1777 S1778 S1779 S1780 S1781 S1782 S1783 S1784 S1785 S1786 S1787 S1788 S1789 S1790 S1791 S1792 S1793 S1794 S1795 S1796 S1797 S1798 S1799 S1800 S1801 S1802 S1803 S1804 S1805 S1806 S1807 S1808 S1809 S1810 S1811 S1812 S1813 S1814 S1815 S1816 S1817 S1818 S1819 S1820 S1821 S1822 S1823 S1824 S1825 S1826 S1827 S1828 S1829 S1830 S1831 S1832 S1833 S1834 S1835 S1836 S1837 S1838 S1839 S1840 S1841 S1842 S1843 S1844 S1845 S1846 S1847 S1848 S1849 S1850 S1851 S1852 S1853 S1854 S1855 S1856 S1857 S1858 S1859 S1860 S1861 S1862 S1863 S1864 S1865 S1866 S1867 S1868 S1869 S1870 S1871 S1872 S1873 S1874 S1875 S1876 S1877 S1878 S1879 S1880 S1881 S1882 S1883 S1884 S1885 S1886 S1887 S1888 S1889 S1890 S1891 S1892 S1893 S1894 S1895 S1896 S1897 S1898 S1899 S1900 S1901 S1902 S1903 S1904 S1905 S1906 S1907 S1908 S1909 S1910 S1911 S1912 S1913 S1914 S1915 S1916 S1917 S1918 S1919 S1920 S1921 S1922 S1923 S1924 S1925 S1926 S1927 S1928 S1929 S1930 S1931 S1932 S1933 S1934 S1935 S1936 S1937 S1938 S1939 S1940 S1941 S1942 S1943 S1944 S1945 S1946 L8 L9 A4
named bodies: "Tv_FrontCover"
